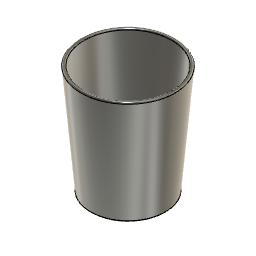
smol_cup (Autodesk Fusion 360 design; units mm, degrees)
Autodesk Fusion 360 part; units mm, degrees
sketch "Sketch1" plane through (0, 0, 0) normal (0, 0, 1) x (1, 0, 0)
  circle A0 centre (0, 0) radius 12.5
  dimension "d1" = 25
  constraint coincident A0.centre origin
  measures "d1" diameter of A0
extrude "Extrude1" add sketch "Sketch1" along normal blind 37 draft 5
shell "Shell1" thickness 1 removed faces 1 at (-7.81, 2.0449, 37)
fillet "Fillet1" radius 0.5 2 edges at (-14.6721, 5.6908, 37) (-13.7362, 5.3278, 37)
fillet "Fillet2" radius 0.5 1 edges at (-11.6541, -4.5202, 0)
